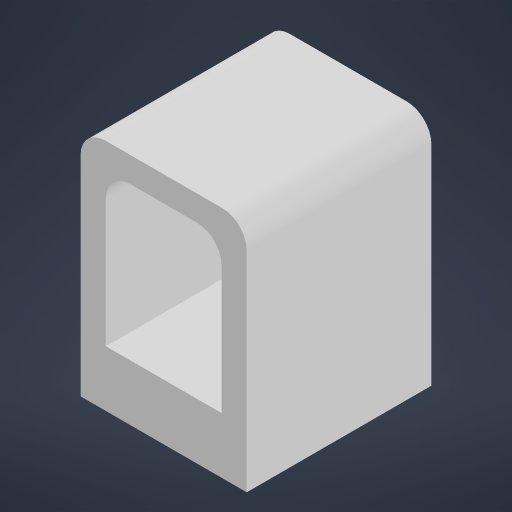
# Autodesk Inventor part: Rod
Saved by Autodesk Inventor 2024.1 (Build 281209000, 209)
## iProperties
Created: 2023-09-06
Part Number: Rod
Material: Generic
Document SubType Name: Modeling
Designer: User
Density: 1 g/cm^3
Appearance: Default
Author: User
Autodesk Inventor part; units mm, degrees
ref_plane "YZ Plane" through (0, 0, 0) normal (1, 0, 0) x (0, 1, 0)
ref_plane "XZ Plane" through (0, 0, 0) normal (0, 1, 0) x (-1, 0, 0)
ref_plane "XY Plane" through (0, 0, 0) normal (0, 0, 1) x (1, 0, 0)
sketch "Sketch1" plane through (0, 0, 0) normal (0, 0, 1) x (1, 0, 0)
  line L0 (0, 0) -> (-13.5, 0)
  line L1 (-13.5, 0) -> (-13.5, 19)
  line L2 (-13.5, 19) -> (0, 19)
  line L3 (0, 19) -> (0, 0)
  dimension "d0" = 13.5
  dimension "d1" = 19
  constraints: 8 end point, 2 parallel, 1 horizontal, 1 perpendicular
  measures "d0" distance of L1.end L2.end
  measures "d1" distance of L0.end L1.end
extrude "Extrusion1" add sketch "Sketch1" along normal blind 10 and the other way blind 5
sketch "Sketch2" plane through (0, 0, 10) normal (0, 0, 1) x (1, 0, 0)
  line L0 (-13.5, 19) -> (-13.5, 0) projected
  line L1 (-13.5, 0) -> (-11.45, 0)
  line L2 (-11.45, 0) -> (-11.45, 4.55)
  line L3 (-11.45, 4.55) -> (-13.5, 4.55)
  line L4 (-13.5, 4.55) -> (-13.5, 0)
  line L5 (0, 19) -> (-13.5, 19) projected
  line L6 (0, 19) -> (-2.05, 19)
  line L7 (-2.05, 19) -> (-2.05, 16.95)
  line L8 (-2.05, 16.95) -> (0, 16.95)
  line L9 (0, 16.95) -> (0, 19)
  line L10 (-11.45, 4.55) -> (-2.05, 4.55)
  line L11 (-2.05, 4.55) -> (-2.05, 16.95)
  line L12 (-2.05, 16.95) -> (-11.45, 16.95)
  line L13 (-11.45, 16.95) -> (-11.45, 4.55)
  point P0 (0, 0)
  dimension "d4" = 2.05
  dimension "d5" = 4.55
  dimension "d6" = 2.05
  dimension "d7" = 2.05
  constraints: 24 end point, 6 parallel, 3 horizontal, 3 perpendicular
  measures "d4" distance of L3.end L2.end
  measures "d5" distance of L2.end L1.end
  measures "d6" distance of L8.end L7.end
  measures "d7" distance of L7.end L6.end
extrude "Extrusion2" cut sketch "Sketch2" against normal blind 10 contours L13 L12 L11 L10
fillet "Fillet1" radius 2 2 edges at (-11.45, 16.95, 5) (-2.05, 16.95, 5)
fillet "Fillet9" radius 2 2 edges at (0, 19, 2.5) (-13.5, 19, 2.5)
body "Solid1"
